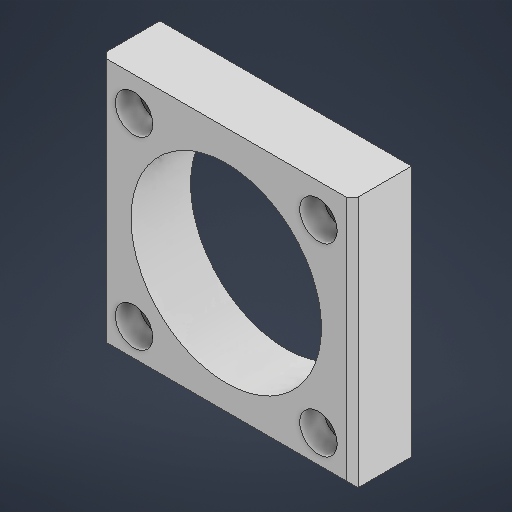
# Autodesk Inventor part: motor_cover
Saved by Autodesk Inventor 2025.1 (Build 291241000, 241)
## iProperties
Created: 2024-12-13
Part Number: motor_cover
Material: Všeobecné
Document SubType Name: Modeling
Designer: lukas
Density: 1 g/cm^3
Appearance: Výchozí
Author: lukas
Autodesk Inventor part; units mm, degrees
ref_plane "YZ Plane" through (0, 0, 0) normal (1, 0, 0) x (0, 1, 0)
ref_plane "XZ Plane" through (0, 0, 0) normal (0, 1, 0) x (-1, 0, 0)
ref_plane "XY Plane" through (0, 0, 0) normal (0, 0, 1) x (1, 0, 0)
sketch "Náčrt1" plane through (0, 0, 0) normal (0, 0, 1) x (1, 0, 0)
  line L0 (0, 29.61) -> (0, -29.61) projected
  line L1 (-29.61, 0) -> (29.61, 0) projected
  line L2 (-21.15, 21.15) -> (21.15, 21.15)
  line L3 (21.15, 21.15) -> (21.15, -21.15)
  line L4 (21.15, -21.15) -> (-21.15, -21.15)
  line L5 (-21.15, -21.15) -> (-21.15, 21.15)
  point P0 (0, 0)
  dimension "d0" = 42.3
  dimension "d1" = 42.3
  constraints: 8 end point, 2 parallel, 1 horizontal, 1 perpendicular, 2 other
  measures "d0" distance of L3.end L4.end
  measures "d1" distance of L2.end L3.end
extrude "Vysunutí1" add sketch "Náčrt1" along normal blind 10
sketch "Náčrt2" plane through (0, 0, 10) normal (0, 0, 1) x (1, 0, 0)
  line L0 (19.15, -19.15) -> (-19.15, -19.15) projected
  line L1 (19.15, 19.15) -> (19.15, -19.15) projected
  line L2 (-19.15, 19.15) -> (19.15, 19.15) projected
  line L3 (-19.15, -19.15) -> (-19.15, 19.15) projected
  point P0 (0, 0)
  point P1 (0, 0)
  constraints: 1 coincident
hole "Díra1" at (0, 0, 10) direction (0, 0, -1) diameter 32 end through all
sketch "Náčrt3" plane through (0, 0, 10) normal (0, 0, 1) x (1, 0, 0)
  circle A0 centre (0, 0) radius 16 projected
  line L0 (-29.61, 0) -> (29.61, 0) projected
  line L1 (0, -29.61) -> (0, 29.61) projected
  point P0 (-15.5, 15.5)
  point P1 (-15.5, -15.5)
  point P2 (15.5, -15.5)
  point P3 (15.5, 15.5)
  dimension "d14" = 31
  dimension "d16" = 31
  constraints: 3 symmetric about line
  measures "d14" distance of point (-15.5, 15.5) point (15.5, 15.5)
  measures "d16" distance of point (15.5, 15.5) point (15.5, -15.5)
hole "Díra2" at (-15.5, 15.5, 10) at (-15.5, -15.5, 10) at (15.5, -15.5, 10) at (15.5, 15.5, 10) direction (0, 0, -1) diameter 3.4 end through all counterbore diameter 6.3 counterbore depth 4 clearance for "Strojní šroub se zápustnou hlavou" size "M3" standard "Ansi M metrický profil"
chamfer "Zkosení2" distance 1 angle 45 3 edges at (21.15, 0, 10) (0, -21.15, 10) (-21.15, 0, 10)
